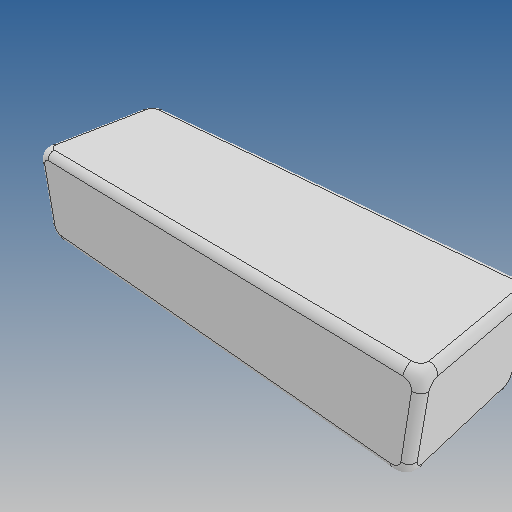
# Autodesk Inventor part: Lipo 3S Battery
Saved by Autodesk Inventor 2026 (Build 300175000, 175)
## iProperties
Created: 2026-07-22
Part Number: Lipo 3S Battery
Material: Generic
Document SubType Name: Modeling
Designer: Pacman Ng
Density: 1 g/cm^3
Appearance: Default
Author: Pacman Ng
Autodesk Inventor part; units mm, degrees
ref_plane "YZ Plane" through (0, 0, 0) normal (1, 0, 0) x (0, 1, 0)
ref_plane "XZ Plane" through (0, 0, 0) normal (0, 1, 0) x (-1, 0, 0)
ref_plane "XY Plane" through (0, 0, 0) normal (0, 0, 1) x (1, 0, 0)
sketch "Sketch2" plane through (0, 0, 0) normal (0, 0, 1) x (1, 0, 0)
  line L0 (-55, 17.5) -> (55, 17.5)
  line L1 (55, 17.5) -> (55, -17.5)
  line L2 (55, -17.5) -> (-55, -17.5)
  line L3 (-55, -17.5) -> (-55, 17.5)
  line L4 (-55, 17.5) -> (55, -17.5) construction
  line L5 (55, 17.5) -> (-55, -17.5) construction
  point P0 (0, 0)
  dimension "d0" = 110
  dimension "d1" = 35
  constraints: 12 end point, 2 midpoint, 2 parallel, 1 horizontal, 1 perpendicular
  measures "d0" distance of L1.end L2.end
  measures "d1" distance of L0.end L1.end
extrude "Extrusion1" add sketch "Sketch2" along normal blind 25
fillet "Fillet1" radius 2 12 edges at (0, -17.5, 25) (-55, 0, 25) (-55, -17.5, 12.5) (-55, 0, 0) (0, -17.5, 0) (55, 0, 25) (55, 17.5, 12.5) (0, 17.5, 25) (0, 17.5, 0) (55, 0, 0) (55, -17.5, 12.5) (-55, 17.5, 12.5)
body "Solid1"
